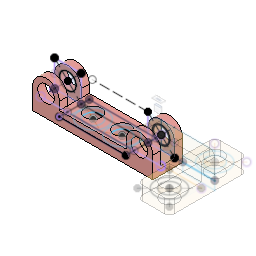
Hinges (Autodesk Fusion 360 design; units mm, degrees)
Autodesk Fusion 360 part; units mm, degrees
note: some values were not read from the file. Chosen so that the rebuilt part matches the saved one: which bodies a step acts on; which face or edge a step refers to. Set by a fixed rule: which sketch regions a step uses.
sketch "Sketch1" plane through (0, 0, 0) normal (0, 0, 1) x (1, 0, 0) in component "HingeCentre"
  line L0 (0, 0) -> (45, 0)
  line L1 (45, 0) -> (45, 166.5146)
  line L2 (45, 166.5146) -> (0, 166.5146)
  line L3 (0, 166.5146) -> (0, 0)
  line L4 (0, 7.9073) -> (45, 7.9073)
  line L5 (45, 7.9073) -> (45, 13.1073)
  line L6 (45, 13.1073) -> (0, 13.1073)
  line L7 (0, 13.1073) -> (0, 7.9073)
  line L8 (0, 13.1073) -> (45, 13.1073)
  line L9 (45, 13.1073) -> (45, 16.1073)
  line L10 (45, 16.1073) -> (0, 16.1073)
  line L11 (0, 16.1073) -> (0, 13.1073)
  line L12 (0, 7.9073) -> (45, 7.9073)
  line L13 (45, 7.9073) -> (45, 4.9073)
  line L14 (45, 4.9073) -> (0, 4.9073)
  line L15 (0, 4.9073) -> (0, 7.9073)
  line L16 (10, 16.1073) -> (10, 4.9073)
  line L17 (35, 16.1073) -> (35, 4.9073)
  dimension "d74" = 45
  dimension "d75" = 5.2
  dimension "d76" = 3
  dimension "d131" = 3
  dimension "d136" = 10
  dimension "d137" = 10
  constraint horizontal L0
  constraint vertical L1
  constraint horizontal L2
  constraint vertical L3
  constraint coincident L0.start L3.end
  constraint horizontal L4
  constraint vertical L5
  constraint horizontal L6
  constraint vertical L7
  constraint coincident L3 L4.start
  constraint horizontal L8
  constraint vertical L9
  constraint horizontal L10
  constraint vertical L11
  constraint horizontal L12
  constraint vertical L13
  constraint horizontal L14
  constraint vertical L15
  constraint coincident L10 L16.start
  constraint coincident L14 L16.end
  constraint perpendicular L14 L16
  constraint coincident L10 L17.start
  constraint perpendicular L10 L17
  constraint coincident L14 L17.end
  measures "d74" distance of L0.start L0.end
  measures "d75" distance of L4.start L6.end
  measures "d76" distance of L6.end L10.end
  measures "d131" distance of L4.start L14.end
  measures "d136" distance of L3 L16
  measures "d137" distance of L1 L17
extrude "Extrude1" add sketch "Sketch1" along normal blind 13 contours L3 L4 L12 L14 L15 L16 | L1 L4 L12 L13 L14 L17 | L3 L6 L8 L10 L11 L16 | L1 L6 L8 L9 L10 L17 makes body 1 at (41.6667, 13.1073, 8.6667) makes body 2 at (3.3333, 7.9073, 8.6667) makes body 3 at (6.6667, 16.1073, 8.6667) makes body 4 at (41.6667, 4.9073, 8.6667) in component "HingeCentre"
extrude "Extrude2" add sketch "Sketch1" along normal blind 3 contours L3 L4 L6 L7 L8 L12 L16 | L4 L12 L14 L16 L17 | L1 L4 L5 L6 L8 L12 L17 | L4 L6 L8 L12 L16 L17 | L6 L8 L10 L16 L17 bodies 1 2 3 4 in component "HingeCentre"
sketch "Sketch2" plane through (0, 13.1073, 0) normal (0, -1, 0) x (1, 0, 0) in component "HingeCentre"
  line L0 (35, 3) -> (45, 3)
  line L1 (45, 3) -> (45, 13)
  line L2 (45, 13) -> (35, 13)
  line L3 (35, 13) -> (45, 3) construction
  line L4 (35, 13) -> (14.1421, 13) construction
  line L5 (35, 3) -> (45, 13) construction
  circle A0 centre (40, 8) radius 3.1
  line L6 (40, 13) -> (40, 3) construction
  circle A1 centre (40, 8) radius 3.1
  line L7 (35, 13) -> (35, 3)
  line L8 (0, 3) -> (10, 3)
  line L9 (10, 3) -> (10, 13)
  line L10 (10, 13) -> (0, 13)
  line L11 (0, 13) -> (0, 3)
  line L12 (0, 13) -> (10, 3) construction
  line L13 (0, 3) -> (10, 13) construction
  circle A2 centre (5, 8) radius 3.1
  dimension "d81" = 45
  dimension "d82" = 90
  dimension "d83" = 6.2
  dimension "d144" = 6.2
  constraint horizontal L4
  constraint coincident L2.end L3.start
  constraint coincident L0 L1.start
  constraint coincident L0.start L5.start
  constraint coincident L4 L1.end
  constraint midpoint L5 A0.centre
  constraint midpoint L2 L6.start
  constraint midpoint L0 L6.end
  constraint symmetric A0 L6 A1
  constraint coincident L10.end L11.start
  constraint coincident L8.end L9.start
  constraint coincident L8.start L11.end
  constraint coincident L9.end L10.start
  constraint midpoint L12 A2.centre
  measures "d81" angle of L3 L4
  measures "d82" angle of L3 L5
  measures "d83" diameter of A0
  measures "d144" diameter of A2
fillet "Fillet1" radius 5 2 edges at (45, 14.6073, 13) (0, 14.6073, 13) on bodies 1 4 in component "HingeCentre"
fillet "Fillet1" radius 5 2 edges at (45, 6.4073, 13) (0, 6.4073, 13) on bodies 1 4 in component "HingeCentre"
fillet "Fillet1" radius 5 4 edges at (35, 14.6073, 13) (10, 14.6073, 13) (10, 6.4073, 13) (35, 6.4073, 13) on bodies 1 4 in component "HingeCentre"
sketch "Sketch3" plane through (0, 0, 0) normal (0, 0, 1) x (1, 0, 0) in component "HingeCentre"
sketch "Sketch1 (2)" plane through (0, 13.1073, 0) normal (0, -1, 0) x (1, 0, 0) in component "HingeLeaver"
  line L0 (35, 3) -> (45, 3)
  circle A0 centre (40, 8) radius 4.8
  line L1 (40.0434, 12.7998) -> (60.0434, 12.7998)
  line L2 (60.0434, 12.7998) -> (60.0434, 3.2002)
  line L3 (60.0434, 3.2002) -> (40.0434, 3.2002)
  line L4 (40.0434, 3.2002) -> (40.0434, 12.7998)
  line L5 (48.0434, 3.2002) -> (60.0434, 3.2002)
  line L6 (60.0434, 3.2002) -> (60.0434, 3)
  line L7 (60.0434, 3) -> (48.0434, 3)
  line L8 (48.0434, 3) -> (48.0434, 3.2002)
  line L9 (48.0434, 3) -> (60.0434, 3)
  line L10 (60.0434, 3) -> (60.0434, 0)
  line L11 (60.0434, 0) -> (48.0434, 0)
  line L12 (48.0434, 0) -> (48.0434, 3)
  line L13 (0, 8) -> (0, 3)
  line L14 (10, 3) -> (10, 8)
  arc A1 (45, 8) -> (35, 8) centre (40, 8) ccw
  line L15 (35, 8) -> (35, 3)
  line L16 (45, 3) -> (45, 8)
  arc A2 (10, 8) -> (0, 8) centre (5, 8) ccw
  line L17 (0, 3) -> (10, 3)
  circle A3 centre (40, 8) radius 3.1
  circle A4 centre (40, 8) radius 3.3
  line L18 (48.0434, 3.2002) -> (60.0434, 3.2002)
  line L19 (60.0434, 3.2002) -> (60.0434, 5.2002)
  line L20 (60.0434, 5.2002) -> (48.0434, 5.2002)
  line L21 (48.0434, 5.2002) -> (48.0434, 3.2002)
  dimension "d129" = 20
  dimension "d130" = 12
  dimension "d145" = 0.2
  dimension "d159" = 2
  constraint horizontal L1
  constraint vertical L2
  constraint horizontal L3
  constraint vertical L4
  constraint coincident A0 L1.start
  constraint coincident A0 L3.end
  constraint horizontal L5
  constraint vertical L6
  constraint horizontal L7
  constraint vertical L8
  constraint coincident L3 L5.start
  constraint horizontal L9
  constraint vertical L10
  constraint horizontal L11
  constraint vertical L12
  constraint coincident L2.end L3.start
  constraint coincident L6.end L7.start
  constraint horizontal L18
  constraint vertical L19
  constraint horizontal L20
  constraint vertical L21
  measures "d129" distance of L1.start L1.end
  measures "d130" distance of L10.end L11.end
  measures "d159" distance of L5.start L20.end
extrude "Extrude1'" add sketch "Sketch1 (2)" along normal blind 5 separate body contours L1 L2 L3 A1 L16 L20 L21 | A0 L1 L3 A1 L16 | L2 L3 L5 L18 L19 L20 L21 | A0 L4 A4 | A0 L4 A4 makes body 5 in component "HingeLeaver"
extrude "Extrude2'" add sketch "Sketch1 (2)" along normal blind 17 contours L2 L3 L5 L18 L19 L20 L21 | L3 L5 L6 L7 L8 L9 L18 | L7 L9 L10 L11 L12 bodies 5 in component "HingeLeaver"
extrude "Extrude3" add sketch "Sketch1 (2)" against normal blind 12 contours L2 L3 L5 L18 L19 L20 L21 | L3 L5 L6 L7 L8 L9 L18 | L7 L9 L10 L11 L12 bodies 5 in component "HingeLeaver"
sketch "Sketch4" plane through (0, 0, 3) normal (0, 0, 1) x (-1, 0, 0) in component "HingeCentre"
  line L0 (-45, -7.9073) -> (-45, -13.1073)
  line L1 (-10, -13.1073) -> (0, -13.1073)
  line L2 (0, -13.1073) -> (0, -7.9073)
  line L3 (-11.6174, -13.1073) -> (-33.3826, -13.1073)
  line L4 (-33.3826, -13.1073) -> (-33.3826, -7.9073)
  line L5 (-33.3826, -7.9073) -> (-11.6174, -7.9073)
  line L6 (-11.6174, -7.9073) -> (-11.6174, -13.1073)
  line L7 (0, -7.9073) -> (-45, -7.9073)
  line L8 (-11.6174, -13.1073) -> (-22.5, -7.9073) construction
  line L9 (-22.5, -7.9073) -> (-33.3826, -13.1073) construction
  circle A0 centre (-27.9413, -10.5073) radius 3.1
  circle A1 centre (-17.0587, -10.5073) radius 3.1
  line L10 (-10, -16.1073) -> (-10, -13.1073)
  line L11 (0, -7.9073) -> (-10, -7.9073)
  line L12 (-10, -7.9073) -> (-10, -4.9073)
  line L13 (-10, -4.9073) -> (-35, -4.9073)
  line L14 (-35, -4.9073) -> (-35, -7.9073)
  line L15 (-35, -7.9073) -> (-45, -7.9073)
  line L16 (-45, -13.1073) -> (-35, -13.1073)
  line L17 (-35, -13.1073) -> (-35, -16.1073)
  line L18 (-35, -16.1073) -> (-10, -16.1073)
  circle A2 centre (-17.0587, -10.5073) radius 5.1
  circle A3 centre (-27.9413, -10.5073) radius 5.1
  line L19 (-10, -16.1073) -> (-35, -16.1073)
  line L20 (-35, -16.1073) -> (-35, -4.9073)
  line L21 (-35, -4.9073) -> (-10, -4.9073)
  line L22 (-10, -4.9073) -> (-10, -16.1073)
  dimension "d99" = 6.2
  dimension "d100" = 6.2
  dimension "d153" = 2
  dimension "d154" = 2
  constraint horizontal L3
  constraint vertical L4
  constraint horizontal L5
  constraint vertical L6
  constraint coincident L1 L3.start
  constraint midpoint L5 L7
  constraint midpoint L7 L8.end
  constraint midpoint L9 A0.centre
  constraint midpoint L8 A1.centre
  constraint horizontal L19
  constraint vertical L20
  constraint horizontal L21
  constraint vertical L22
  constraint coincident L13.end L14.start
  constraint coincident L10.start L18.end
  measures "d99" diameter of A0
  measures "d100" diameter of A1
extrude "Extrude4" cut sketch "Sketch4" against normal up to surface (3 mm away) contours L5 L7 A0 | L3 L5 L7 A0 | L3 A0 | L5 L7 A1 | L3 L5 L7 A1 | L3 A1 bodies 1 in component "HingeCentre"
sketch "Sketch2 (2)" plane through (0, 0, 3.2002) normal (0, 0, 1) x (-1, 0, 0) in component "HingeLeaver"
  line L0 (-48.0434, -8.1073) -> (-48.0434, 3.8927)
  line L1 (-48.0434, 3.8927) -> (-60.0434, 3.8927)
  line L2 (-60.0434, 3.8927) -> (-60.0434, -8.1073)
  line L3 (-60.0434, -8.1073) -> (-48.0434, -8.1073)
  line L4 (-48.0434, -8.1073) -> (-60.0434, 3.8927) construction
  line L5 (-48.0434, 3.8927) -> (-60.0434, -8.1073) construction
  line L6 (-48.0434, -25.1073) -> (-60.0434, -13.1073) construction
  line L7 (-48.0434, -13.1073) -> (-60.0434, -25.1073) construction
  circle A0 centre (-54.0434, -19.1073) radius 3.1
  circle A1 centre (-54.0434, -2.1073) radius 3.1
  circle A2 centre (-54.0434, -2.1073) radius 5.1
  circle A3 centre (-54.0434, -19.1073) radius 5.1
  point P0 (-60.0434, -8.1073)
  point P1 (-60.0434, -13.1073)
  point P2 (-48.0434, -13.1073)
  point P3 (-48.0434, -25.1073)
  point P4 (-60.0434, -25.1073)
  dimension "d117" = 6.2
  dimension "d118" = 6.2
  dimension "d147" = 2
  dimension "d148" = 2
  constraint coincident L0.start L3.end
  constraint coincident L1.end L2.start
  constraint coincident L0.end L1.start
  constraint coincident P0 L2.end
  constraint coincident P1 L6.end
  constraint coincident P2 L7.start
  constraint midpoint L6 A0.centre
  constraint midpoint L4 A1.centre
  measures "d117" diameter of A0
  measures "d118" diameter of A1
extrude "Extrude5" cut sketch "Sketch2 (2)" along normal up to surface (-3.2002 mm away) and the other way up to surface (-2 mm away) contours A0 | A1 bodies 5 in component "HingeLeaver"
fillet "Fillet5" radius 2 4 edges at (48.0434, -3.8927, 2.6001) (60.0434, -3.8927, 2.6001) (60.0434, 25.1073, 2.6001) (48.0434, 25.1073, 2.6001) on bodies 5 in component "HingeLeaver"
fillet "Fillet6" radius 2 1 edges at (60.0434, 10.6073, 12.7998) on bodies 5 in component "HingeLeaver"
extrude "Extrude5'" cut sketch "Sketch2" along normal up to surface (8.2 mm away) and the other way up to surface (3 mm away) contours A0 A1 | A2 bodies 1 in component "HingeCentre"
extrude "Extrude7" add sketch "Sketch4" along normal blind 2 contours L5 L7 L12 L13 L14 A2 A3 L20 L21 L22 | L3 L4 L6 L7 L10 L17 L18 A2 A3 L19 L20 L22 | L3 L4 L5 L7 A3 | L5 L7 A0 A3 | L3 L5 L7 A0 A3 | L3 A0 A3 | L3 L5 L7 A0 A3 | L3 L5 L7 A2 A3 | L5 L7 A1 A2 | L3 L5 L7 A1 A2 | L3 L5 L6 L7 A2 | L3 A1 A2 | L3 L5 L7 A1 A2 bodies 1 in component "HingeCentre"
extrude "Extrude6" [suppressed] in component "HingeCentre"
extrude "Extrude6'" [suppressed] in component "HingeLeaver"
component "HingeCentre" placed x (1, 0, 0) y (0, 1, 0) z (0, 0, 1) at (0, 0, 0)
component "HingeLeaver" placed x (1, 0, 0) y (0, 1, 0) z (0, 0, 1) at (0, 0, 0)
equation "d83 = deuvelHole"
equation "d99 = deuvelHole"
equation "d100 = deuvelHole"
equation "d117 = deuvelHole"
equation "d118 = deuvelHole"
equation "d144 = deuvelHole"
equation "deuvelHole = 6.2 mm"
